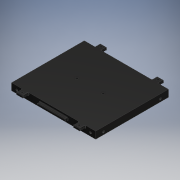
# Autodesk Inventor part: Structure_+Z
Saved by Autodesk Inventor 2018 (Build 220112000, 112)
## iProperties
Created: 2018-07-04
Part Number: Structure_+Z
Material: Aluminum 6061
Document SubType Name: Modeling
Designer: Bradley
Density: 2.7 g/cm^3
Appearance: Anodized - Dark Gray
Mass: 173.922 g
Surface Area: 203.124 cm^2
Volume: 64.4155 cm^3
Author: Bradley
Autodesk Inventor part; units mm, degrees
ref_plane "YZ Plane" through (0, 0, 0) normal (1, 0, 0) x (0, 1, 0)
ref_plane "XZ Plane" through (0, 0, 0) normal (0, 1, 0) x (-1, 0, 0)
ref_plane "XY Plane" through (0, 0, 0) normal (0, 0, 1) x (1, 0, 0)
sketch "Sketch1" plane through (0, 0, 0) normal (0, 0, 1) x (1, 0, 0)
  line L0 (48, -41.5) -> (48, 41.5)
  line L1 (48, 41.5) -> (36.5, 41.5)
  line L2 (36.5, 41.5) -> (36.5, 48)
  line L3 (36.5, 48) -> (28.5, 48)
  line L4 (28.5, 48) -> (28.5, 41.5)
  line L5 (28.5, 41.5) -> (-28.5, 41.5)
  line L6 (-28.5, 41.5) -> (-28.5, 48)
  line L7 (-28.5, 48) -> (-36.5, 48)
  line L8 (-36.5, 48) -> (-36.5, 41.5)
  line L9 (-36.5, 41.5) -> (-48, 41.5)
  line L10 (-48, 41.5) -> (-48, -41.5)
  line L11 (-48, -41.5) -> (-36.5, -41.5)
  line L12 (-36.5, -41.5) -> (-36.5, -48)
  line L13 (-36.5, -48) -> (-28.5, -48)
  line L14 (-28.5, -48) -> (-28.5, -41.5)
  line L15 (-28.5, -41.5) -> (28.5, -41.5)
  line L16 (28.5, -48) -> (36.5, -48)
  line L17 (36.5, -41.5) -> (36.5, -48)
  line L18 (28.5, -48) -> (28.5, -41.5)
  line L19 (36.5, -41.5) -> (48, -41.5)
  line L20 (32.5, 45) -> (-32.5, 45) construction
  line L21 (-32.5, 45) -> (-32.5, -45) construction
  line L22 (-32.5, -45) -> (32.5, -45) construction
  line L23 (32.5, -45) -> (32.5, 45) construction
  line L24 (32.5, 45) -> (-32.5, -45) construction
  line L25 (-32.5, 45) -> (32.5, -45) construction
  circle A0 centre (-32.5, -45) radius 3 construction
  point P0 (0, 0)
  point P1 (-48, 0)
  point P2 (0, -41.5)
  point P3 (-32.5, -48)
  point P4 (-32.5, 48)
  point P5 (32.5, -48)
  point P6 (32.5, 48)
  dimension "d0" = 83
  dimension "d2" = 65
  dimension "d3" = 90
  dimension "d4" = 6
  dimension "d5" = 6.5
  dimension "d6" = 8
  dimension "d7" = 96
  constraints: 52 end point, 20 point on line, 12 perpendicular, 8 midpoint, 3 collinear, 3 parallel, 1 centre point, 1 coincident, 1 horizontal, 1 horizontal alignment, 1 vertical, 1 vertical alignment
  measures "d0" distance of L9.end L10.end
  measures "d2" distance of L22.end L21.end
  measures "d3" distance of L21.end L20.end
  measures "d4" diameter of A0
  measures "d5" distance of L13.end L14.end
  measures "d6" distance of L12.end L13.end
  measures "d7" distance between parallel lines of L10 L0
extrude "Extrusion1" add sketch "Sketch1" along normal mid plane 8
sketch "Sketch2" plane through (0, 0, 4) normal (0, 0, 1) x (1, 0, 0)
  line L0 (32.5, 45) -> (-32.5, 45) construction
  line L1 (-32.5, -45) -> (32.5, -45) construction
  line L2 (-15, 0) -> (15, 0) construction
  point P0 (0, 0)
  point P1 (0, 0)
  dimension "d10" = 30
  constraints: 7 coincident, 2 end point, 1 horizontal, 1 midpoint
  measures "d10" distance of L2.start L2.end
hole "Hole1" at (-32.5, 45, 4) at (32.5, 45, 4) at (15, 0, 4) at (-15, 0, 4) at (-32.5, -45, 4) at (32.5, -45, 4) direction (0, 0, -1) diameter 2.621 end through all thread size "M3x0.35" class "6H" standard "ANSI Metric M Profile"
sketch "Sketch3" plane through (0, 0, -4) normal (0, 0, -1) x (-1, 0, 0)
  circle A0 centre (32.5, -45) radius 1.3105 projected
  circle A1 centre (-15, 0) radius 1.3105 projected
  circle A2 centre (32.5, 45) radius 1.3105 projected
  circle A3 centre (-32.5, 45) radius 1.3105 projected
  circle A4 centre (15, 0) radius 1.3105 projected
  circle A5 centre (-32.5, -45) radius 1.3105 projected
  line L0 (-48, 41.5) -> (-48, -41.5) projected
  line L1 (-48, -41.5) -> (-36.5, -41.5) projected
  line L2 (-36.5, -41.5) -> (-36.5, -48) projected
  line L3 (-36.5, -48) -> (-28.5, -48) projected
  line L4 (-28.5, -48) -> (-28.5, -41.5) projected
  line L5 (-28.5, -41.5) -> (28.5, -41.5) projected
  line L6 (28.5, -41.5) -> (28.5, -48) projected
  line L7 (28.5, -48) -> (36.5, -48) projected
  line L8 (36.5, -48) -> (36.5, -41.5) projected
  line L9 (36.5, -41.5) -> (48, -41.5) projected
  line L10 (48, -41.5) -> (48, 41.5) projected
  line L11 (48, 41.5) -> (36.5, 41.5) projected
  line L12 (36.5, 41.5) -> (36.5, 48) projected
  line L13 (36.5, 48) -> (28.5, 48) projected
  line L14 (28.5, 48) -> (28.5, 41.5) projected
  line L15 (28.5, 41.5) -> (-28.5, 41.5) projected
  line L16 (-28.5, 41.5) -> (-28.5, 48) projected
  line L17 (-28.5, 48) -> (-36.5, 48) projected
  line L18 (-36.5, 48) -> (-36.5, 41.5) projected
  line L19 (-36.5, 41.5) -> (-48, 41.5) projected
  line L20 (-36.5, -41.5) -> (-36.5, -48) projected
  line L21 (-36.5, -41.5) -> (-28.5, -41.5)
  line L22 (-36.5, 48) -> (-36.5, 41.5) projected
  line L23 (-36.5, 41.5) -> (-28.5, 41.5)
  line L24 (28.5, 48) -> (28.5, 41.5) projected
  line L25 (28.5, 41.5) -> (36.5, 41.5)
  line L26 (36.5, -41.5) -> (48, -41.5) projected
  line L27 (36.5, -41.5) -> (28.5, -41.5)
  point P0 (0, 0)
  constraints: 8 end point, 3 perpendicular, 1 collinear
extrude "Extrusion2" cut sketch "Sketch3" against normal blind 5 contours L18 L17 L16 L23 | L21 L4 L3 L2 | L14 L13 L12 L25 | L27 L8 L7 L6
sketch "Sketch4" plane through (-48, -41.5, -4) normal (0, -1, 0) x (1, 0, 0)
  line L0 (11.5, 5) -> (11.5, 8) projected
  line L1 (0, 8) -> (11.5, 8) projected
  line L2 (0, 0) -> (0, 8) projected
  line L3 (96, 0) -> (0, 0) projected
  line L4 (96, 8) -> (96, 0) projected
  line L5 (84.5, 8) -> (96, 8) projected
  line L6 (84.5, 5) -> (84.5, 8) projected
  line L7 (84.5, 5) -> (76.5, 5) projected
  line L8 (76.5, 5) -> (76.5, 8) projected
  line L9 (19.5, 8) -> (76.5, 8) projected
  line L10 (19.5, 5) -> (19.5, 8) projected
  line L11 (19.5, 5) -> (11.5, 5) projected
  line L12 (63, 4) -> (33, 4) construction
  line L13 (63, 5.5) -> (33, 5.5)
  line L14 (33, 2.5) -> (63, 2.5)
  arc A0 (63, 2.5) -> (63, 5.5) centre (63, 4) ccw
  arc A1 (33, 5.5) -> (33, 2.5) centre (33, 4) ccw
  point P0 (48, 4)
  dimension "d40" = 30
  dimension "d41" = 3
  constraints: 8 end point, 4 point on circle, 4 tangent, 2 centre point, 2 parallel, 1 midpoint
  measures "d40" distance of L12.start L12.end
  measures "d41" distance between parallel lines of L13 L14
extrude "Extrusion3" add sketch "Sketch4" along normal blind 3 contours A0 L14 A1 L13
mirror "Mirror1" about plane through (0, 0, 0) normal (0, 1, 0) of "Extrusion3"
fillet "Fillet1" radius 1 16 edges at (-36.5, -44.75, 1) (-28.5, -44.75, 4) (-28.5, -44.75, 1) (28.5, -44.75, 4) (28.5, -44.75, 1) (36.5, -44.75, 4) (36.5, -44.75, 1) (36.5, 44.75, 4) (36.5, 44.75, 1) (28.5, 44.75, 1) (28.5, 44.75, 4) (-36.5, 44.75, 1) (-36.5, 44.75, 4) (-28.5, 44.75, 1) (-28.5, 44.75, 4) (-36.5, -44.75, 4)
chamfer "Chamfer1" distance 0.5 angle 45 40 edges at (28.7929, 48, 3.7071) (28.5, 48, 2.5) (28.7929, 48, 1.2929) (32.5, 48, 1) (36.2071, 48, 1.2929) (36.5, 48, 2.5) (36.2071, 48, 3.7071) (32.5, 48, 4) (-32.5, 48, 4) (-36.2071, 48, 3.7071) (-36.5, 48, 2.5) (-36.2071, 48, 1.2929) (-32.5, 48, 1) (-28.7929, 48, 1.2929) (-28.5, 48, 2.5) (-28.7929, 48, 3.7071) (32.5, -48, 4) (36.2071, -48, 3.7071) (36.5, -48, 2.5) (36.2071, -48, 1.2929) (32.5, -48, 1) (28.7929, -48, 1.2929) (28.5, -48, 2.5) (28.7929, -48, 3.7071) (-36.5, -48, 2.5) (-36.2071, -48, 3.7071) (-32.5, -48, 4) (-28.7929, -48, 3.7071) (-28.5, -48, 2.5) (-28.7929, -48, 1.2929) (-32.5, -48, 1) (-36.2071, -48, 1.2929) (0, -44.5, 1.5) (-16.5, -44.5, 0) (0, -44.5, -1.5) (16.5, -44.5, 0) (0, 44.5, 1.5) (-16.5, 44.5, 0) (0, 44.5, -1.5) (16.5, 44.5, 0)
fillet "Fillet2" radius 0.381 36 edges at (-36.2071, -41.5, 3.7071) (-36.2071, -41.5, 1.2929) (-32.5, -41.5, 1) (-28.7929, -41.5, 1.2929) (-28.5, -41.5, 2.5) (-28.7929, -41.5, 3.7071) (-36.5, -41.5, 2.5) (32.5, -41.5, 1) (36.2071, -41.5, 1.2929) (36.5, -41.5, 2.5) (36.2071, -41.5, 3.7071) (28.5, -41.5, 2.5) (28.7929, -41.5, 3.7071) (28.7929, -41.5, 1.2929) (28.5, 41.5, 2.5) (28.7929, 41.5, 1.2929) (32.5, 41.5, 1) (36.2071, 41.5, 1.2929) (36.5, 41.5, 2.5) (36.2071, 41.5, 3.7071) (28.7929, 41.5, 3.7071) (-36.5, 41.5, 2.5) (-36.2071, 41.5, 1.2929) (-32.5, 41.5, 1) (-28.7929, 41.5, 1.2929) (-28.5, 41.5, 2.5) (-28.7929, 41.5, 3.7071) (-36.2071, 41.5, 3.7071) (0, -41.5, -1.5) (-16.5, -41.5, 0) (0, -41.5, 1.5) (16.5, -41.5, 0) (16.5, 41.5, 0) (0, 41.5, 1.5) (-16.5, 41.5, 0) (0, 41.5, -1.5)
sketch "Sketch5" plane through (-48, -41.5, -4) normal (0, -1, 0) x (1, 0, 0)
  arc A0 (84.881, 7) -> (84.4524, 8) centre (83.5, 7) ccw projected
  line L0 (84.881, 6) -> (84.881, 7) projected
  arc A1 (83.5, 4.619) -> (84.881, 6) centre (83.5, 6) ccw projected
  line L1 (77.5, 4.619) -> (83.5, 4.619) projected
  arc A2 (76.119, 6) -> (77.5, 4.619) centre (77.5, 6) ccw projected
  line L2 (76.119, 7) -> (76.119, 6) projected
  arc A3 (76.5476, 8) -> (76.119, 7) centre (77.5, 7) ccw projected
  line L3 (19.4524, 8) -> (76.5476, 8) projected
  arc A4 (19.881, 7) -> (19.4524, 8) centre (18.5, 7) ccw projected
  line L4 (19.881, 6) -> (19.881, 7) projected
  arc A5 (18.5, 4.619) -> (19.881, 6) centre (18.5, 6) ccw projected
  line L5 (12.5, 4.619) -> (18.5, 4.619) projected
  arc A6 (11.119, 6) -> (12.5, 4.619) centre (12.5, 6) ccw projected
  line L6 (11.119, 7) -> (11.119, 6) projected
  arc A7 (11.5476, 8) -> (11.119, 7) centre (12.5, 7) ccw projected
  line L7 (0, 8) -> (11.5476, 8) projected
  line L8 (0, 0) -> (0, 8) projected
  line L9 (96, 0) -> (0, 0) projected
  line L10 (96, 8) -> (96, 0) projected
  line L11 (84.4524, 8) -> (96, 8) projected
  line L12 (6, 3.5) -> (90, 3.5) construction
  point P0 (48, 3.5)
  point P1 (48, 0)
  dimension "d31" = 84
  dimension "d60" = 4.5
  constraints: 2 coincident, 2 end point, 2 midpoint, 1 horizontal, 1 vertical alignment
  measures "d31" distance of L12.start L12.end
  measures "d60" distance between parallel lines of L12 L7
hole "Hole2" at (-42, -41.5, -0.5) at (42, -41.5, -0.5) direction (0, 1, 0) diameter 2.459 depth 8.8 tip angle 118 thread size "M3x0.5" class "6H" standard "ANSI Metric M Profile"
mirror "Mirror2" about plane through (0, 0, 0) normal (0, 1, 0) of "Hole2"
sketch "Sketch6" plane through (48, -41.5, 4) normal (1, 0, 0) x (0, 0, -1)
  line L0 (8, 83) -> (0, 83) projected
  line L1 (0, 0) -> (0, 83) projected
  line L2 (0, 0) -> (8, 0) projected
  line L3 (8, 83) -> (8, 0) projected
  line L4 (5, 9) -> (5, 74) construction
  line L5 (8, 0) -> (8, 83) projected
  point P0 (5, 41.5)
  point P1 (8, 41.5)
  dimension "d42" = 65
  dimension "d50" = 5
  constraints: 2 coincident, 2 end point, 2 midpoint, 1 horizontal alignment, 1 vertical
  measures "d42" distance of L4.start L4.end
  measures "d50" distance between parallel lines of L4 L1
hole "Hole3" at (48, -32.5, -1) at (48, 32.5, -1) direction (-1, 0, 0) diameter 2.621 depth 8.1 tip angle 118 thread size "M3x0.35" class "6H" standard "ANSI Metric M Profile"
mirror "Mirror3" about plane through (0, 0, 0) normal (1, 0, 0) of "Hole3"
body "Solid1"
